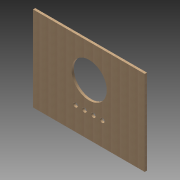
# Autodesk Inventor part: Base
Saved by Autodesk Inventor 2015 (Build 190159000, 159)
## iProperties
Created: 2015-01-25
Part Number: Base
Material: Generic
Document SubType Name: Modeling
Designer: Michael7
Density: 1 g/cm^3
Appearance: White Ash
Author: Michael7
Autodesk Inventor part; units mm, degrees
ref_plane "YZ Plane" through (0, 0, 0) normal (1, 0, 0) x (0, 1, 0)
ref_plane "XZ Plane" through (0, 0, 0) normal (0, 1, 0) x (-1, 0, 0)
ref_plane "XY Plane" through (0, 0, 0) normal (0, 0, 1) x (1, 0, 0)
sketch "Sketch1" plane through (0, 0, 0) normal (0, 0, 1) x (1, 0, 0)
  line L0 (-317.5, 241.3) -> (0, 241.3)
  line L1 (0, 241.3) -> (0, 0)
  line L2 (0, 0) -> (-317.5, 0)
  line L3 (-317.5, 0) -> (-317.5, 241.3)
  dimension "d0" = 317.5
  dimension "d1" = 241.3
  constraints: 8 end point, 2 parallel, 1 horizontal, 1 perpendicular
  measures "d0" distance of L0.start L0.end
  measures "d1" distance of L0.end L1.end
extrude "Extrusion1" add sketch "Sketch1" along normal blind 6.35
sketch "Sketch2" plane through (0, 0, 6.35) normal (0, 0, 1) x (1, 0, 0)
  circle A0 centre (-120.65, 66.675) radius 6.35
  line L0 (-317.5, 0) -> (0, 0) projected
  line L1 (0, 0) -> (0, 241.3) projected
  circle A1 centre (-196.85, 66.675) radius 6.35
  line L2 (-317.5, 241.3) -> (-317.5, 0) projected
  circle A2 centre (-171.45, 66.675) radius 6.35
  circle A3 centre (-146.05, 66.675) radius 6.35
  dimension "d4" = 12.7
  dimension "d5" = 66.675
  dimension "d7" = 12.7
  dimension "d8" = 66.675
  dimension "d10" = 12.7
  dimension "d11" = 12.7
  dimension "d12" = 66.675
  dimension "d13" = 66.675
  dimension "d20" = 114.3
  dimension "d21" = 114.3
  dimension "d26" = 12.7
  dimension "d27" = 12.7
  constraints: 4 centre point
  measures "d4" diameter of A0
  measures "d5" distance from line of L0 A0.centre
  measures "d7" diameter of A1
  measures "d8" distance from line of L0 A1.centre
  measures "d10" diameter of A3
  measures "d11" diameter of A2
  measures "d12" distance from line of L0 A2.centre
  measures "d13" distance from line of L0 A3.centre
  measures "d20" distance edge to line of A1 L2
  measures "d21" distance edge to line of A0 L1
extrude "Extrusion2" cut sketch "Sketch2" against normal blind 6.35
sketch "Sketch3" plane through (0, 0, 6.35) normal (0, 0, 1) x (1, 0, 0)
  circle A0 centre (-157.9499, 146.8501) radius 49.9999
  line L0 (0, 0) -> (0, 241.3) projected
  line L1 (0, 241.3) -> (-317.5, 241.3) projected
  dimension "d28" = 99.9998
  dimension "d29" = 107.95
  dimension "d30" = 44.45
  constraints: 1 centre point
  measures "d28" diameter of A0
  measures "d29" distance edge to line of A0 L0
  measures "d30" distance edge to line of A0 L1
extrude "Extrusion3" cut sketch "Sketch3" against normal blind 6.35
body "Solid1"
